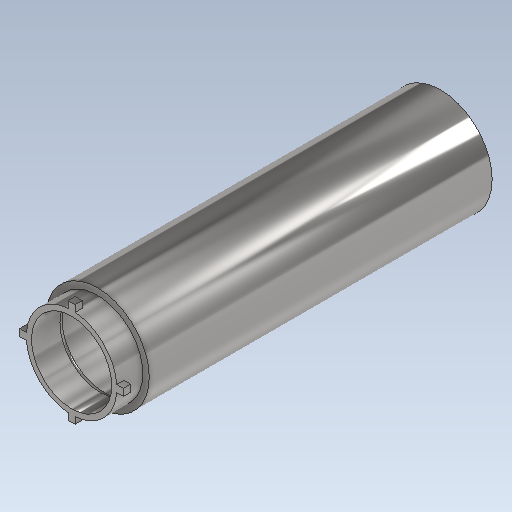
# Autodesk Inventor part: HERRAMIENTA_p2
Saved by Autodesk Inventor 2026 (Build 300175000, 175)
## iProperties
Created: 2026-07-16
Part Number: HERRAMIENTA_p2
Material: Plástico PET
Document SubType Name: Sheet Metal
Designer: User
Density: 1.541 g/cm^3
Sheet Metal Rule: Por defecto_mm
Appearance: Acero - Pulido
Author: User
Autodesk Inventor part; units mm, degrees
note: some values were not read from the file. Chosen so that the rebuilt part matches the saved one: edges of "Empalme2".
ref_plane "YZ Plane" through (0, 0, 0) normal (1, 0, 0) x (0, 1, 0)
ref_plane "XZ Plane" through (0, 0, 0) normal (0, 1, 0) x (-1, 0, 0)
ref_plane "XY Plane" through (0, 0, 0) normal (0, 0, 1) x (1, 0, 0)
sketch "Boceto1" plane through (0, 0, 0) normal (0, 0, 1) x (1, 0, 0)
  circle A0 centre (0, 0) radius 15
  dimension "d0" = 30
  constraints: 1 centre point, 1 coincident
  measures "d0" diameter of A0
extrude "Extrusión1" add sketch "Boceto1" along normal blind 145.5
sketch "Boceto2" plane through (0, 0, 145.5) normal (0, 0, 1) x (1, 0, 0)
  circle A0 centre (0, 0) radius 12.5
  circle A1 centre (0, 0) radius 15
  dimension "d5" = 25
  constraints: 2 centre point, 1 coincident
  measures "d5" diameter of A0
extrude "Extrusión2" cut sketch "Boceto2" against normal blind 10
sketch "Boceto3" plane through (0, 0, 145.5) normal (0, 0, 1) x (1, 0, 0)
  circle A0 centre (0, 0) radius 10
  dimension "d8" = 20
  constraints: 1 centre point, 1 coincident
  measures "d8" diameter of A0
extrude "Extrusión3" cut sketch "Boceto3" against normal blind 145.5
sketch "Boceto4" plane through (0, 0, 145.5) normal (0, 0, 1) x (1, 0, 0)
  circle A0 centre (0, 0) radius 15
  circle A1 centre (0, 0) radius 12.5 projected
  line L0 (-14.9345, 1.4) -> (-12.4214, 1.4)
  line L1 (-12.4214, 1.4) -> (-12.4214, -1.4)
  line L2 (-12.4214, -1.4) -> (-14.9345, -1.4)
  line L3 (-15.0786, 1.4) -> (-12.4214, -1.4) construction
  line L4 (-12.4214, 1.4) -> (-14.9469, -1.2612) construction
  line L5 (-1.4, -14.9345) -> (-1.4, -12.4214)
  line L6 (-1.4, -12.4214) -> (1.4, -12.4214)
  line L7 (1.4, -12.4214) -> (1.4, -14.9345)
  line L8 (-1.4, -15.0786) -> (1.4, -12.4214) construction
  line L9 (-1.4, -12.4214) -> (1.2612, -14.9469) construction
  line L10 (14.9345, -1.4) -> (12.4214, -1.4)
  line L11 (12.4214, -1.4) -> (12.4214, 1.4)
  line L12 (12.4214, 1.4) -> (14.9345, 1.4)
  line L13 (15.0786, -1.4) -> (12.4214, 1.4) construction
  line L14 (12.4214, -1.4) -> (14.9469, 1.2612) construction
  line L15 (1.4, 14.9345) -> (1.4, 12.4214)
  line L16 (1.4, 12.4214) -> (-1.4, 12.4214)
  line L17 (-1.4, 12.4214) -> (-1.4, 14.9345)
  line L18 (1.4, 15.0786) -> (-1.4, 12.4214) construction
  line L19 (1.4, 12.4214) -> (-1.2612, 14.9469) construction
  point P0 (-13.75, 0)
  point P1 (0, -13.75)
  point P2 (13.75, 0)
  point P3 (0, 13.75)
  dimension "d12" = 2.8
  dimension "d15" = 360
  constraints: 40 end point, 4 point on line, 3 point on circle, 1 centre point, 1 coincident, 1 horizontal, 1 midpoint, 1 parallel, 1 perpendicular, 51 other
  measures "d12" distance of L0.end L1.end
extrude "Extrusión4" add sketch "Boceto4" against normal blind 2.8 contours A0 L10 A1 L12 | L15 A1 L17 A0 | A0 L5 A1 L7 | L0 A1 L2 A0
sketch "Boceto5" plane through (0, 0, 0) normal (0, 0, -1) x (-1, 0, 0)
  circle A0 centre (0, 0) radius 12.5
  circle A1 centre (0, 0) radius 10
  constraints: 2 centre point, 2 coincident
extrude "Extrusión5" cut sketch "Boceto5" against normal blind 133
fillet "Empalme1" radius 2.5 1 edges at (12.5, 0, 133)
sketch "Boceto6" plane through (0, 0, 0) normal (0, 0, -1) x (-1, 0, 0)
  circle A0 centre (0, 0) radius 12.5 projected
  circle A1 centre (0, 0) radius 12.5
  circle A2 centre (0, 0) radius 10.925
  dimension "d22" = 21.85
  constraints: 2 centre point, 2 coincident
  measures "d22" diameter of A2
extrude "Extrusión6" add sketch "Boceto6" against normal blind 5
sketch "Boceto7" plane through (0, 0, 0) normal (0, 0, -1) x (-1, 0, 0)
  circle A0 centre (0, 0) radius 17.5
  circle A1 centre (0, 0) radius 15
  dimension "d25" = 35
  dimension "d28" = 30
  constraints: 2 centre point, 2 coincident
  measures "d25" diameter of A0
  measures "d28" diameter of A1
extrude "Extrusión7" add sketch "Boceto7" against normal blind 135.5
sketch "Boceto9" plane through (0, 0, 0) normal (0, 0, -1) x (-1, 0, 0)
  circle A0 centre (0, 0) radius 16.5
  dimension "d29" = 33
  constraints: 1 centre point, 1 coincident
  measures "d29" diameter of A0
extrude "Extrusión8" cut sketch "Boceto9" against normal blind 135.5
sketch "Boceto10" plane through (0, 0, 0) normal (0, 0, -1) x (-1, 0, 0)
  circle A0 centre (0, 0) radius 16.5
  circle A1 centre (0, 0) radius 10.925
  dimension "d32" = 21.85
  constraints: 2 centre point, 2 coincident
  measures "d32" diameter of A1
extrude "Extrusión9" add sketch "Boceto10" against normal blind 5
sketch "Boceto11" plane through (0, 0, 0) normal (0, 0, -1) x (-1, 0, 0)
  circle A0 centre (0, 0) radius 17.5 projected
  circle A1 centre (0, 0) radius 20
  circle A2 centre (0, 0) radius 17.5
  dimension "d35" = 40
  dimension "d36" = 35
  constraints: 2 centre point, 2 coincident
  measures "d35" diameter of A1
  measures "d36" diameter of A2
extrude "Extrusión10" add sketch "Boceto11" against normal blind 135.5
sketch "Boceto12" plane through (0, 0, 135.5) normal (0, 0, 1) x (1, 0, 0)
  circle A0 centre (0, 0) radius 17.5
  circle A1 centre (0, 0) radius 16.5
  dimension "d39" = 35
  constraints: 2 centre point, 2 coincident
  measures "d39" diameter of A0
extrude "Extrusión11" cut sketch "Boceto12" against normal blind 134
sketch "Boceto13" plane through (0, 0, 145.5) normal (0, 0, 1) x (1, 0, 0)
  circle A0 centre (0, 0) radius 15.5
  circle A1 centre (0, 0) radius 17.5
  dimension "d42" = 31
  constraints: 2 centre point, 2 coincident
  measures "d42" diameter of A0
extrude "Extrusión12" cut sketch "Boceto13" against normal blind 10 contours A0
sketch "Boceto14" plane through (0, 0, 135.5) normal (0, 0, 1) x (1, 0, 0)
  circle A0 centre (0, 0) radius 17.5
  circle A1 centre (0, 0) radius 15.5
  dimension "d45" = 31
  constraints: 2 centre point, 2 coincident
  measures "d45" diameter of A1
extrude "Extrusión13" add sketch "Boceto14" along normal blind 10
sketch "Boceto15" plane through (0, 0, 145.5) normal (0, 0, 1) x (1, 0, 0)
  line L0 (-20, 1.375) -> (-16.4197, 1.375)
  line L1 (-16.4426, -1.375) -> (-20, -1.375)
  line L2 (-20, -1.375) -> (-20, 1.375)
  circle A0 centre (0, 0) radius 17.5 projected
  line L3 (-16.4197, 1.375) -> (-16.4426, -1.375)
  circle A1 centre (0, 0) radius 16.5 projected
  line L4 (-1.375, -20) -> (-1.375, -16.4197)
  line L5 (1.375, -16.4426) -> (1.375, -20)
  line L6 (1.375, -20) -> (-1.375, -20)
  line L7 (-1.375, -16.4197) -> (1.375, -16.4426)
  line L8 (20, -1.375) -> (16.4197, -1.375)
  line L9 (16.4426, 1.375) -> (20, 1.375)
  line L10 (20, 1.375) -> (20, -1.375)
  line L11 (16.4197, -1.375) -> (16.4426, 1.375)
  line L12 (1.375, 20) -> (1.375, 16.4197)
  line L13 (-1.375, 16.4426) -> (-1.375, 20)
  line L14 (-1.375, 20) -> (1.375, 20)
  line L15 (1.375, 16.4197) -> (-1.375, 16.4426)
  point P0 (-17.5, 0)
  point P1 (0, -17.5)
  point P2 (17.5, 0)
  point P3 (0, 17.5)
  dimension "d52" = 360
  constraints: 32 end point, 1 horizontal, 1 horizontal alignment, 1 parallel, 40 other
extrude "Extrusión14" add sketch "Boceto15" against normal blind 2.75 contours L0 A0 L1 L2 | L0 A1 L1 A0 | L0 L3 A1 | L13 L14 L12 A0 | A0 L12 A1 L13 | A1 L12 L15 | L4 A1 L5 A0 | A0 L5 L6 L4 | L4 L7 A1 | L9 L10 L8 A0 | A0 L8 A1 L9 | A1 L8 L11
sketch "Boceto16" plane through (0, 0, 0) normal (0, 0, -1) x (-1, 0, 0)
  circle A0 centre (0, 0) radius 20 projected
  circle A1 centre (0, 0) radius 10.925 projected
extrude "Extrusión15" cut sketch "Boceto16" against normal blind 1
sketch "Boceto17" plane through (0, 0, 1) normal (0, 0, -1) x (-1, 0, 0)
  circle A0 centre (0, 0) radius 17.5
  dimension "d58" = 35
  constraints: 1 centre point, 1 coincident
  measures "d58" diameter of A0
extrude "Extrusión16" cut sketch "Boceto17" against normal blind 20
sketch "Boceto18" plane through (0, 0, 1) normal (0, 0, -1) x (-1, 0, 0)
  circle A0 centre (0, 0) radius 17.5
  circle A1 centre (0, 0) radius 10.925
  dimension "d61" = 21.85
  dimension "d62" = 35
  constraints: 2 centre point, 2 coincident
  measures "d61" diameter of A1
  measures "d62" diameter of A0
extrude "Extrusión17" add sketch "Boceto18" against normal blind 5
sketch "Boceto19" plane through (0, 0, 1) normal (0, 0, -1) x (-1, 0, 0)
  circle A0 centre (0, 0) radius 10.925 projected
  circle A1 centre (0, 0) radius 20 projected
extrude "Extrusión18" cut sketch "Boceto19" against normal blind 2
thicken "Engrosado1" operation add thickness 1 both sides no extend neighbours no toward (-0.9870503, 0.1604113, 0) faces at (17.2734, -2.8072, 92.3333) (16.5137, -2.6325, 135.5)
fillet "Empalme2" radius 2 1 edges at (-16.5, 0, 134.5)
equation "\"Radio_pliegue\" = Grosor"
equation "\"Anchura_desahogo_plegado\" = Grosor"
equation "\"Profundidad_desahogo_plegado\" = 0.5 * Grosor"
equation "\"Tamaño_destalonado\" = 4 * Grosor"
equation "\"Remanente_mínimo\" = 2 * Grosor"
equation "\"Radiodetransición\" = Radio_pliegue"
equation "\"Tamaño_de_radio_de_Jacobi\" = Radio_pliegue"
equation "\"TamañoSeparación\" = Grosor"
equation "\"Grosor\" = 0.5"
